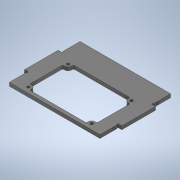
# Autodesk Inventor part: Cockpit_bottom_frame
Saved by Autodesk Inventor 2020.4 (Build 244396000, 396)
## iProperties
Created: 2022-01-06
Part Number: Cockpit_bottom_frame
Material: アセタール樹脂、黒
Document SubType Name: Modeling
Designer: Masato Kubotera
Density: 1.425 g/cm^3
Appearance: 滑らか - 黒
Mass: 58.9249 g
Surface Area: 211.38 cm^2
Volume: 41.3508 cm^3
Description: POM T5
Author: Masato Kubotera
Autodesk Inventor part; units mm, degrees
ref_plane "YZ Plane" through (0, 0, 0) normal (1, 0, 0) x (0, 1, 0)
ref_plane "XZ Plane" through (0, 0, 0) normal (0, 1, 0) x (-1, 0, 0)
derived "Cockpit_side_frame.ipt"
sketch "スケッチ1" plane through (0, 0, 0) normal (0, 1, 0) x (-1, 0, 0)
  line L0 (-60, 36.75) -> (60, 36.75) construction
  line L1 (60, 36.75) -> (60, -36.75) construction
  line L2 (60, -36.75) -> (-60, -36.75) construction
  line L3 (-60, -36.75) -> (-60, 36.75) construction
  line L4 (-60, 36.75) -> (60, -36.75) construction
  line L5 (60, 36.75) -> (-60, -36.75) construction
  line L6 (-52.5, 6.75) -> (52.5, 6.75) construction
  line L7 (52.5, 6.75) -> (52.5, 1.75) construction
  line L8 (52.5, 1.75) -> (-52.5, 1.75) construction
  line L9 (-52.5, 1.75) -> (-52.5, 6.75) construction
  line L10 (-52.5, 6.75) -> (52.5, 1.75) construction
  line L11 (52.5, 6.75) -> (-52.5, 1.75) construction
  line L12 (0, 36.75) -> (0, -36.75) construction
  line L13 (-57.5, 34.25) -> (-52.5, 34.25) construction
  line L14 (-52.5, 34.25) -> (-52.5, -34.25) construction
  line L15 (-52.5, -34.25) -> (-57.5, -34.25) construction
  line L16 (-57.5, -34.25) -> (-57.5, 34.25) construction
  line L17 (-57.5, 34.25) -> (-52.5, -34.25) construction
  line L18 (-52.5, 34.25) -> (-57.5, -34.25) construction
  line L19 (-55, 36.75) -> (-60, 31.75)
  line L20 (-60, 0) -> (60, 0) construction
  line L21 (-46.5, 41.75) -> (32.5, 41.75) construction
  line L22 (32.5, 41.75) -> (32.5, 11.75) construction
  line L23 (32.5, 11.75) -> (-46.5, 11.75) construction
  line L24 (-46.5, 11.75) -> (-46.5, 41.75) construction
  line L25 (-46.5, 41.75) -> (32.5, 11.75) construction
  line L26 (32.5, 41.75) -> (-46.5, 11.75) construction
  line L27 (-55, -36.75) -> (-60, -31.75)
  line L28 (-60, 31.75) -> (-60, -31.75)
  line L29 (55, -36.75) -> (60, -31.75)
  line L30 (-52.5, -29.25) -> (52.5, -29.25) construction
  line L31 (52.5, -29.25) -> (52.5, -34.25) construction
  line L32 (52.5, -34.25) -> (-52.5, -34.25) construction
  line L33 (-52.5, -34.25) -> (-52.5, -29.25) construction
  line L34 (-52.5, -29.25) -> (52.5, -34.25) construction
  line L35 (52.5, -29.25) -> (-52.5, -34.25) construction
  line L36 (-25, -29.25) -> (-25, -34.25) construction
  line L37 (-55, -34.25) -> (-55, 34.25) construction
  line L38 (-57.5, 12.5) -> (-52.5, 12.5) construction
  line L39 (-57.55, 12.55) -> (-52.45, 12.55)
  line L40 (-52.45, 12.55) -> (-52.45, -12.55)
  line L41 (-52.45, -12.55) -> (-57.55, -12.55)
  line L42 (-57.55, -12.55) -> (-57.55, 12.55)
  line L43 (-57.55, 12.55) -> (-52.45, -12.55) construction
  line L44 (-52.45, 12.55) -> (-57.55, -12.55) construction
  arc A0 (-52.45, 11.0651) -> (-53.9349, 12.55) centre (-53.1925, 11.8075) ccw
  circle A1 centre (-55, 20) radius 1.6
  circle A2 centre (-55, -20) radius 1.6
  arc A3 (-53.9349, -12.55) -> (-52.45, -11.0651) centre (-53.1925, -11.8075) ccw
  line L45 (-57.5, -12.5) -> (-52.5, -12.5) construction
  arc A4 (-56.0651, 12.55) -> (-57.55, 11.0651) centre (-56.8075, 11.8075) ccw
  arc A5 (-57.55, -11.0651) -> (-56.0651, -12.55) centre (-56.8075, -11.8075) ccw
  line L46 (-52.5, -31.75) -> (52.5, -31.75) construction
  line L47 (-25.05, -34.25) -> (-25.05, -29.2)
  line L48 (-25.05, -29.2) -> (25.05, -29.2)
  circle A6 centre (-32.5, -31.75) radius 1.6
  circle A7 centre (32.5, -31.75) radius 1.6
  line L49 (25, -29.25) -> (25, -34.25) construction
  line L50 (52.5, 36.75) -> (57.5, 36.75) construction
  line L51 (57.5, 36.75) -> (57.5, -34.25) construction
  line L52 (57.5, -34.25) -> (52.5, -34.25) construction
  line L53 (52.5, -34.25) -> (52.5, 36.75) construction
  line L54 (52.5, 36.75) -> (57.5, -34.25) construction
  line L55 (57.5, 36.75) -> (52.5, -34.25) construction
  line L56 (52.5, 1.25) -> (57.5, 1.25) construction
  line L57 (52.5, -11.25) -> (57.5, -11.25) construction
  line L58 (55, -34.25) -> (55, 36.75) construction
  circle A8 centre (55, -18.75) radius 1.6
  line L59 (60, -11.3) -> (52.45, -11.3)
  line L60 (52.45, -11.3) -> (52.45, 13.8)
  arc A9 (52.45, -9.8151) -> (53.9349, -11.3) centre (53.1925, -10.5575) ccw
  line L61 (60, 13.8) -> (52.45, 13.8)
  arc A10 (53.9349, 13.8) -> (52.45, 12.3151) centre (53.1925, 13.0575) ccw
  line L62 (52.5, 13.75) -> (57.5, 13.75) construction
  circle A11 centre (55, 21.25) radius 1.6
  arc A12 (-23.5651, -29.2) -> (-25.05, -30.6849) centre (-24.3075, -29.9425) ccw
  arc A13 (25.05, -30.6849) -> (23.5651, -29.2) centre (24.3075, -29.9425) ccw
  circle A14 centre (-55, 20) radius 3
  circle A15 centre (-32.5, -31.75) radius 3
  circle A16 centre (-55, -20) radius 3
  circle A17 centre (32.5, -31.75) radius 3
  line L63 (-25.05, -34.25) -> (-27.55, -36.75)
  line L64 (-55, -36.75) -> (-27.55, -36.75)
  line L65 (25.05, -34.25) -> (27.55, -36.75)
  line L66 (25.05, -34.25) -> (25.05, -29.2)
  line L67 (55, -36.75) -> (27.55, -36.75)
  line L68 (25.05, 6.8) -> (-25.05, 6.8)
  line L69 (-25.05, 6.8) -> (-25.05, 1.7)
  line L70 (-25.05, 1.7) -> (25.05, 1.7)
  line L71 (25.05, 1.7) -> (25.05, 6.8)
  line L72 (25.05, 6.8) -> (-25.05, 1.7) construction
  line L73 (-25.05, 6.8) -> (25.05, 1.7) construction
  line L74 (-25, 6.75) -> (-25, 1.75) construction
  arc A18 (-23.5651, 6.8) -> (-25.05, 5.3151) centre (-24.3075, 6.0575) ccw
  line L75 (52.5, 4.25) -> (-52.5, 4.25) construction
  circle A19 centre (-32.5, 4.25) radius 1.6
  line L76 (25, 6.75) -> (25, 1.75) construction
  arc A20 (25.05, 5.3151) -> (23.5651, 6.8) centre (24.3075, 6.0575) ccw
  circle A21 centre (32.5, 4.25) radius 1.6
  arc A22 (-25.05, 3.1849) -> (-23.5651, 1.7) centre (-24.3075, 2.4425) ccw
  arc A23 (23.5651, 1.7) -> (25.05, 3.1849) centre (24.3075, 2.4425) ccw
  line L77 (60, 31.75) -> (60, 13.8)
  line L78 (60, -11.3) -> (60, -31.75)
  circle A24 centre (-32.5, 4.25) radius 3
  circle A25 centre (55, -18.75) radius 3
  circle A26 centre (55, 21.25) radius 3
  circle A27 centre (32.5, 4.25) radius 3
  line L79 (60, 31.75) -> (60, 36.75)
  line L80 (21, 36.75) -> (-55, 36.75)
  line L81 (60, 36.75) -> (55, 41.75)
  line L82 (55, 41.75) -> (50, 41.75)
  line L83 (50, 41.75) -> (50, 36.75)
  line L84 (50, 36.75) -> (40.5, 36.75)
  line L85 (40.5, 36.75) -> (40.5, 41.75)
  line L86 (40.5, 41.75) -> (30.5, 41.75)
  line L87 (30.5, 41.75) -> (30.5, 36.75)
  line L88 (30.5, 36.75) -> (21, 36.75)
  line L89 (21, 36.75) -> (21, 36.75)
  circle A28 centre (-45, 4.25) radius 1.75
  line L90 (35.5, 41.75) -> (35.5, 36.75) construction
  line L91 (37.9, -8.6) -> (47.1, -8.6) construction
  line L92 (47.1, -8.6) -> (47.1, -22.4) construction
  line L93 (47.1, -22.4) -> (37.9, -22.4) construction
  line L94 (37.9, -22.4) -> (37.9, -8.6) construction
  line L95 (37.9, -8.6) -> (47.1, -22.4) construction
  line L96 (47.1, -8.6) -> (37.9, -22.4) construction
  line L97 (37.2, -7.95) -> (47.8, -7.95) construction
  line L98 (47.8, -7.95) -> (47.8, -23.05) construction
  line L99 (47.8, -23.05) -> (37.2, -23.05) construction
  line L100 (37.2, -23.05) -> (37.2, -7.95) construction
  line L101 (37.2, -7.95) -> (47.8, -23.05) construction
  line L102 (47.8, -7.95) -> (37.2, -23.05) construction
  line L103 (42.5, -7.95) -> (42.5, -23.05) construction
  line L104 (47.8, -15.5) -> (37.2, -15.5) construction
  line L105 (38.6349, -7.9) -> (46.3651, -7.9)
  line L106 (37.15, -9.3849) -> (37.15, -21.6151)
  line L107 (39.3349, -8.55) -> (45.6651, -8.55)
  line L108 (37.85, -10.0349) -> (37.85, -20.9651)
  arc A29 (38.6349, -7.9) -> (37.15, -9.3849) centre (37.8925, -8.6425) ccw
  arc A30 (39.3349, -8.55) -> (37.85, -10.0349) centre (38.5925, -9.2925) ccw
  arc A31 (47.85, -9.3849) -> (46.3651, -7.9) centre (47.1075, -8.6425) ccw
  arc A32 (47.15, -10.0349) -> (45.6651, -8.55) centre (46.4075, -9.2925) ccw
  line L109 (38.6349, -23.1) -> (46.3651, -23.1)
  line L110 (39.3349, -22.45) -> (45.6651, -22.45)
  arc A33 (37.85, -20.9651) -> (39.3349, -22.45) centre (38.5925, -21.7075) ccw
  arc A34 (37.15, -21.6151) -> (38.6349, -23.1) centre (37.8925, -22.3575) ccw
  arc A35 (46.3651, -23.1) -> (47.85, -21.6151) centre (47.1075, -22.3575) ccw
  arc A36 (45.6651, -22.45) -> (47.15, -20.9651) centre (46.4075, -21.7075) ccw
  line L111 (47.15, -10.0349) -> (47.15, -20.9651)
  line L112 (47.85, -9.3849) -> (47.85, -21.6151)
  line L113 (-45.5, -4.25) -> (10.5, -4.25)
  line L114 (12.5, -6.25) -> (12.5, -22.25)
  line L115 (10.5, -24.25) -> (-45.5, -24.25)
  line L116 (-47.5, -22.25) -> (-47.5, -6.25)
  line L117 (-47.5, -4.25) -> (12.5, -24.25) construction
  line L118 (12.5, -4.25) -> (-47.5, -24.25) construction
  arc A37 (-45.5, -4.25) -> (-47.5, -6.25) centre (-45.5, -6.25) ccw
  arc A38 (-47.5, -22.25) -> (-45.5, -24.25) centre (-45.5, -22.25) ccw
  arc A39 (10.5, -24.25) -> (12.5, -22.25) centre (10.5, -22.25) ccw
  arc A40 (12.5, -6.25) -> (10.5, -4.25) centre (10.5, -6.25) ccw
  line L119 (26.5, 36.75) -> (26.5, 32.75) construction
  line L120 (24.5, 32.75) -> (28.5, 32.75) construction
  line L121 (28.5, 32.75) -> (28.5, 36.75) construction
  line L122 (24.5, 32.75) -> (24.5, 36.75) construction
  line L123 (42.5, 32.75) -> (42.5, 36.75) construction
  line L124 (44.5, 36.75) -> (44.5, 32.75) construction
  line L125 (46.5, 32.75) -> (42.5, 32.75) construction
  line L126 (46.5, 32.75) -> (46.5, 36.75) construction
  arc A41 (48.5151, 36.75) -> (50, 38.2349) centre (49.2575, 37.4925) ccw
  arc A42 (29.0151, 36.75) -> (30.5, 38.2349) centre (29.7575, 37.4925) ccw
  arc A43 (40.5, 38.2349) -> (41.9849, 36.75) centre (41.2425, 37.4925) ccw
  line L127 (30.5, 36.75) -> (40.5, 36.75)
  point P0 (0, 0)
  point P1 (0, 4.25)
  point P2 (-55, 0)
  point P3 (-55, 0)
  point P4 (-7, 26.75)
  point P5 (0, -31.75)
  point P6 (0, 4.25)
  point P7 (42.5, -15.5)
  point P8 (37.15, -7.9)
  point P9 (37.85, -8.55)
  point P10 (-17.5, -14.25)
  dimension "d2" = 34.25
  dimension "d3" = 105
  dimension "d4" = 50
  dimension "d5" = 65
  measures "d2" vertical distance of L32.end L20.start
  measures "d3" distance of L31.end L32.end
  measures "d4" distance between parallel lines of L49 L36
  measures "d5" distance of A7.centre A6.centre
ref_plane "作業平面1" through (0, 0, -34.25) normal (0, 0, 1) x (1, 0, 0)
sketch "スケッチ2" plane through (0, 0, -34.25) normal (0, 0, 1) x (1, 0, 0)
  line L0 (52.5, -134.5) -> (52.5, 0)
  line L1 (-52.5, 0) -> (-52.5, -134.5)
  line L2 (-52.5, -134.5) -> (52.5, 0) construction
  line L3 (52.5, -134.5) -> (-52.5, 0) construction
  line L4 (-25, 0) -> (-25, 5)
  line L5 (-25, 5) -> (25, 5)
  line L6 (0, -139.5) -> (0, 5) construction
  line L7 (-52.5, -67.25) -> (52.5, -67.25) construction
  arc A0 (-27.1, 0) -> (-25, 0) centre (-26.05, 0) ccw
  line L8 (25, 0) -> (25, 5)
  arc A1 (25, 0) -> (27.1, 0) centre (26.05, 0) ccw
  line L9 (-25, -134.5) -> (-25, -139.5)
  line L10 (-25, -139.5) -> (25, -139.5)
  arc A2 (-25, -134.5) -> (-27.1, -134.5) centre (-26.05, -134.5) ccw
  line L11 (25, -134.5) -> (25, -139.5)
  arc A3 (27.1, -134.5) -> (25, -134.5) centre (26.05, -134.5) ccw
  line L12 (-52.5, 0) -> (-27.1, 0)
  line L13 (52.5, 0) -> (27.1, 0)
  line L14 (-52.5, -134.5) -> (-27.1, -134.5)
  line L15 (52.5, -134.5) -> (27.1, -134.5)
  line L16 (47.5, -17.25) -> (-17.5, -17.25) construction
  line L17 (-17.5, -17.25) -> (-17.5, -117.25) construction
  line L18 (-17.5, -117.25) -> (47.5, -117.25) construction
  line L19 (47.5, -117.25) -> (47.5, -17.25) construction
  line L20 (47.5, -17.25) -> (-17.5, -117.25) construction
  line L21 (-17.5, -17.25) -> (47.5, -117.25) construction
  circle A4 centre (44.5, -20.25) radius 2
  line L22 (-14.5, -114.25) -> (44.5, -114.25) construction
  line L23 (44.5, -114.25) -> (44.5, -20.25) construction
  line L24 (44.5, -20.25) -> (-14.5, -20.25) construction
  line L25 (-14.5, -20.25) -> (-14.5, -114.25) construction
  line L26 (-14.5, -114.25) -> (44.5, -20.25) construction
  line L27 (44.5, -114.25) -> (-14.5, -20.25) construction
  line L28 (15, -17.25) -> (15, -117.25) construction
  circle A5 centre (44.5, -114.25) radius 2
  circle A6 centre (-14.5, -20.25) radius 2
  circle A7 centre (-14.5, -114.25) radius 2
  arc A8 (40.5, -17.25) -> (47.5, -24.25) centre (44.5, -20.25) ccw
  arc A9 (47.5, -110.25) -> (40.5, -117.25) centre (44.5, -114.25) ccw
  arc A10 (-17.5, -24.25) -> (-10.5, -17.25) centre (-14.5, -20.25) ccw
  arc A11 (-10.5, -117.25) -> (-17.5, -110.25) centre (-14.5, -114.25) ccw
  line L29 (40.5, -17.25) -> (-10.5, -17.25)
  line L30 (-17.5, -24.25) -> (-17.5, -110.25)
  line L31 (-10.5, -117.25) -> (40.5, -117.25)
  line L32 (47.5, -110.25) -> (47.5, -24.25)
  circle A12 centre (44.5, -20.25) radius 3 construction
  circle A13 centre (44.5, -114.25) radius 3 construction
  circle A14 centre (-14.5, -20.25) radius 3 construction
  circle A15 centre (-14.5, -114.25) radius 3 construction
  point P0 (0, 0)
  point P1 (0, -67.25)
  point P2 (0, -67.25)
  point P3 (15, -67.25)
  dimension "d6" = 105
  dimension "d7" = 134.5
  dimension "d8" = 50
  dimension "d9" = 1.05
  dimension "d11" = 5
  dimension "d21" = 65
  dimension "d22" = 100
  dimension "d23" = 5
  dimension "d24" = 4
  dimension "d25" = 3
  dimension "d26" = 3
  dimension "d27" = 5
  dimension "d29" = 6
  constraints: 66 end point, 27 symmetric about line, 16 centre point, 16 point on circle, 14 midpoint, 6 perpendicular, 6 point on line, 5 parallel, 3 coincident, 3 collinear, 3 horizontal, 1 tangent, 1 vertical, 12 other
  measures "d6" distance of L1.end L0.start
  measures "d7" distance of L1.start L1.end
  measures "d8" distance of L5.end L4.end
  measures "d9" radius of A0
  measures "d11" distance from line of L4.start L5
  measures "d21" distance of L18.end L17.end
  measures "d22" distance of L17.end L16.end
  measures "d23" horizontal distance of L16.start L0.end
  measures "d24" diameter of A4
  measures "d25" horizontal distance of L23.end L16.start
  measures "d26" horizontal distance of L16.start L23.end
  measures "d27" radius of A8
  measures "d29" diameter of A12
extrude "押し出し1" add sketch "スケッチ2" along normal blind 5
hole "穴1" at (32.5, 0, -31.75) at (-32.5, 0, -31.75) direction (0, -1, 0) diameter 3.242 depth 6 tip angle 118 thread size "M4x0.7" class "6H" standard "ISO Metric profile"
fillet "フィレット1" radius 2 8 edges at (47.5, -110.25, -31.75) (40.5, -117.25, -31.75) (-10.5, -117.25, -31.75) (-17.5, -110.25, -31.75) (47.5, -24.25, -31.75) (40.5, -17.25, -31.75) (-10.5, -17.25, -31.75) (-17.5, -24.25, -31.75)
equation "\"d6\" = d3"
equation "\"d8\" = d4"
equation "\"d26\" = d25"
equation "\"d1\" = -d2"
